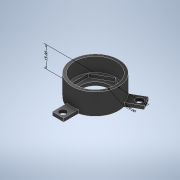
# Autodesk Inventor part: receptor_manguera
Saved by Autodesk Inventor 2022 (Build 260153000, 153)
## iProperties
Created: 2022-04-19
Part Number: receptor_manguera
Material: Generic
Document SubType Name: Modeling
Designer: ferna
Density: 1 g/cm^3
Appearance: Glossy - Black
Author: ferna
Autodesk Inventor part; units mm, degrees
ref_plane "YZ Plane" through (0, 0, 0) normal (1, 0, 0) x (0, 1, 0)
ref_plane "XZ Plane" through (0, 0, 0) normal (0, 1, 0) x (-1, 0, 0)
ref_plane "XY Plane" through (0, 0, 0) normal (0, 0, 1) x (1, 0, 0)
sketch "Sketch1" plane through (0, 0, 0) normal (0, 1, 0) x (-1, 0, 0)
  line L0 (12.25, -7.0725) -> (0, -14.1451)
  line L1 (0, -14.1451) -> (-12.25, -7.0725)
  line L2 (-12.25, -7.0725) -> (-12.25, 7.0725)
  line L3 (-12.25, 7.0725) -> (0, 14.1451)
  line L4 (0, 14.1451) -> (12.25, 7.0725)
  line L5 (12.25, 7.0725) -> (12.25, -7.0725)
  circle A0 centre (0, 0) radius 16.5
  dimension "d0" = 12.25
  dimension "d1" = 33
  constraints: 12 end point, 2 coincident, 1 centre point, 13 other
  measures "d0" distance from line of L5 point (0, 0)
  measures "d1" diameter of A0
extrude "Extrusion1" add sketch "Sketch1" along normal blind 5
sketch "Sketch2" plane through (0, 0, 0) normal (0, -1, 0) x (1, 0, 0)
  line L0 (0, 14.1451) -> (-12.25, 7.0725) projected
  line L1 (-12.25, 7.0725) -> (-12.25, -7.0725) projected
  line L2 (-12.25, -7.0725) -> (0, -14.1451) projected
  line L3 (0, -14.1451) -> (12.25, -7.0725) projected
  line L4 (12.25, -7.0725) -> (12.25, 7.0725) projected
  line L5 (12.25, 7.0725) -> (0, 14.1451) projected
  point P0 (0, 0)
extrude "Extrusion2" add sketch "Sketch2" against normal blind 2.5
sketch "Sketch3" plane through (0, 0, 0) normal (0, -1, 0) x (1, 0, 0)
  circle A0 centre (0, 0) radius 10
  dimension "d6" = 20
  constraints: 1 centre point, 1 coincident
  measures "d6" diameter of A0
extrude "Extrusion3" cut sketch "Sketch3" against normal blind 2.5
sketch "Sketch4" plane through (0, 5, 0) normal (0, 1, 0) x (1, 0, 0)
  circle A0 centre (0, 0) radius 14.5
  circle A1 centre (0, 0) radius 16.5 projected
  dimension "d9" = 29
  constraints: 1 centre point, 1 coincident
  measures "d9" diameter of A0
extrude "Extrusion4" add sketch "Sketch4" along normal blind 10
sketch "Sketch5" plane through (0, 0, 0) normal (0, -1, 0) x (1, 0, 0)
  circle A0 centre (0, 0) radius 16.5 projected
  arc A1 (14.2894, -8.25) -> (0, 16.5) centre (0, 0) ccw
  line L0 (0, 0) -> (14.2894, -8.25) construction
  line L1 (0, 0) -> (0, 16.5) construction
  arc A2 (0, 16.5) -> (-14.2894, -8.25) centre (0, 0) ccw
  line L2 (0, 0) -> (-14.2894, -8.25) construction
  line L3 (0, 0) -> (0, 16.5) construction
  circle A3 centre (0, 0) radius 14.5 projected
  line L4 (0, 14.5) -> (4, 14.5)
  line L5 (4, 14.5) -> (4, 26.5)
  line L6 (4, 26.5) -> (-4, 26.5)
  line L7 (0, 14.5) -> (-4, 14.5)
  line L8 (-4, 14.5) -> (-4, 26.5)
  line L9 (0, 16.5) -> (0, 23)
  circle A4 centre (0, 23) radius 2.5
  line L10 (-12.5574, -7.25) -> (-10.5574, -10.7141)
  line L11 (-12.5574, -7.25) -> (-14.5574, -3.7859)
  line L12 (-14.2894, -8.25) -> (-19.9186, -11.5)
  line L13 (-10.5574, -10.7141) -> (-20.9497, -16.7141)
  circle A5 centre (-19.9186, -11.5) radius 2.5
  line L14 (-24.9497, -9.7859) -> (-20.9497, -16.7141)
  line L15 (-14.5574, -3.7859) -> (-24.9497, -9.7859)
  line L16 (12.5574, -7.25) -> (14.5574, -3.7859)
  line L17 (12.5574, -7.25) -> (10.5574, -10.7141)
  line L18 (14.2894, -8.25) -> (19.9186, -11.5)
  line L19 (14.5574, -3.7859) -> (24.9497, -9.7859)
  circle A6 centre (19.9186, -11.5) radius 2.5
  line L20 (20.9497, -16.7141) -> (24.9497, -9.7859)
  line L21 (10.5574, -10.7141) -> (20.9497, -16.7141)
  point P0 (11.8632, -11.468)
  point P1 (15.8632, -4.5398)
  point P2 (-15.8632, -4.5398)
  point P3 (-11.8632, -11.468)
  point P4 (4, 16.0078)
  point P5 (-4, 16.0078)
  dimension "d12" = 120
  dimension "d13" = 120
  dimension "d14" = 4
  dimension "d15" = 12
  dimension "d16" = 8
  dimension "d17" = 4
  dimension "d18" = 6.5
  dimension "d19" = 5
  dimension "d22" = 360
  constraints: 44 end point, 5 centre point, 5 coincident, 5 point on circle, 5 point on line, 2 horizontal, 2 perpendicular, 1 vertical alignment, 47 other
  measures "d12" angle of L0 L1
  measures "d13" angle of L3 L2
  measures "d14" distance of L4.start L4.end
  measures "d15" distance of L4.end L5.end
  measures "d16" distance of L5.end L6.end
  measures "d17" distance of L4.start L7.end
  measures "d18" distance of L1.end L9.end
  measures "d19" diameter of A4
extrude "Extrusion5" add sketch "Sketch5" against normal blind 2.5 contours A0 L8 L6 L5 | L19 L20 L21 A0 | A0 L13 L14 L15
body "Solid1"
